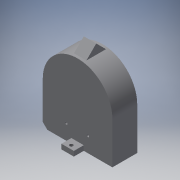
# Autodesk Inventor part: Tail2
Saved by Autodesk Inventor 2016 (Build 200138000, 138)
## iProperties
Created: 2017-03-09
Part Number: Tail2
Material: Generic
Document SubType Name: Modeling
Designer: Owner
Density: 1 g/cm^3
Appearance: Default
Author: Owner
Autodesk Inventor part; units mm, degrees
ref_plane "YZ Plane" through (0, 0, 0) normal (1, 0, 0) x (0, 1, 0)
ref_plane "XZ Plane" through (0, 0, 0) normal (0, 1, 0) x (-1, 0, 0)
sketch "Sketch1" plane through (0, 0, 0) normal (0, 0, 1) x (1, 0, 0)
  line L0 (6.35, -26.3445) -> (6.35, -31.3445) projected
  line L1 (6.35, -31.3445) -> (38.1, -31.3445) projected
  line L2 (38.1, -31.3445) -> (38.1, 11.7555) projected
  arc A0 (38.1, 11.7555) -> (-38.1, 11.7555) centre (0, 11.7555) ccw projected
  line L3 (-38.1, 11.7555) -> (-38.1, -31.3445) projected
  line L4 (-38.1, -31.3445) -> (-6.35, -31.3445) projected
  line L5 (-6.35, -31.3445) -> (-6.35, -26.3445) projected
  line L6 (-6.35, -26.3445) -> (6.35, -26.3445) projected
  circle A1 centre (0, 11.7555) radius 35.56
  line L7 (-35.56, 11.7555) -> (33.02, 11.7555)
  line L8 (33.02, -31.3445) -> (-35.56, -31.3445)
  line L9 (-35.56, -31.3445) -> (-35.56, 11.7555)
  line L10 (35.56, 11.7555) -> (-35.56, 11.7555)
  line L11 (-35.56, 11.7555) -> (-35.56, -31.3445)
  line L12 (-35.56, -31.3445) -> (35.56, -31.3445)
  line L13 (35.56, -31.3445) -> (35.56, 11.7555)
  point P0 (0, 0)
  dimension "d0" = 71.12
  constraints: 14 end point, 3 parallel, 2 horizontal, 2 point on circle, 1 centre point, 1 coincident, 1 perpendicular, 1 point on line
  measures "d0" diameter of A1
extrude "Extrusion1" add sketch "Sketch1" along normal blind 25.4 contours L6 L5 L4 L9 A1 L13 L1 L0 | L0 L8 L5 L6 | L10 L7 A1 | A1 L7 L10
sketch "Sketch2" plane through (0, 0, 0) normal (0, 0, -1) x (-1, 0, 0)
  line L0 (6.3749, -31.3445) -> (-6.9601, -31.3445) projected
  line L1 (-6.9601, -31.3445) -> (-6.9601, -26.3445) projected
  line L2 (-6.9601, -26.3445) -> (6.3749, -26.3445) projected
  line L3 (6.3749, -26.3445) -> (6.3749, -31.3445) projected
  line L4 (35.56, -31.3445) -> (-35.56, -31.3445) projected
  line L5 (0, -26.3445) -> (6.35, -26.3445)
  line L6 (6.35, -26.3445) -> (-6.35, -26.3445)
  line L7 (-6.35, -26.3445) -> (6.35, -26.3445)
  line L8 (6.35, -26.3445) -> (6.35, -21.3445)
  line L9 (6.35, -21.3445) -> (-6.35, -21.3445)
  line L10 (-6.35, -21.3445) -> (-6.35, -26.3445)
  line L11 (-6.35, -26.3445) -> (-6.35, -21.3445)
  point P0 (0, 0)
  dimension "d45" = 6.35
  dimension "d46" = 12.7
  dimension "d51" = 12.7
  constraints: 14 end point, 3 equal length, 1 horizontal, 1 perpendicular
  measures "d45" distance of L5.start L5.end
  measures "d46" distance of L5.end L6.end
  measures "d51" distance between parallel lines of L8 L10
extrude "Extrusion2" add sketch "Sketch2" along normal blind 10.16 contours L2 L10 L9 L8
sketch "Sketch4" plane through (0, 0, 25.4) normal (0, 0, 1) x (1, 0, 0)
  line L0 (-35.56, -31.3445) -> (35.56, -31.3445) projected
  line L1 (-35.56, -31.3445) -> (35.56, -31.3445)
  line L2 (0, -31.3445) -> (6.35, -31.3445)
  line L3 (6.35, -31.3445) -> (-6.35, -31.3445)
  line L4 (6.9601, -26.3445) -> (-6.35, -26.3445) projected
  line L5 (-6.35, -31.3445) -> (6.35, -31.3445)
  line L6 (6.35, -31.3445) -> (6.35, -26.3445)
  line L7 (6.35, -26.3445) -> (-6.35, -26.3445)
  line L8 (-6.35, -26.3445) -> (-6.35, -31.3445)
  point P0 (0, 0)
  dimension "d39" = 6.35
  dimension "d40" = 12.7
  dimension "d52" = 12.7
  constraints: 14 end point, 3 point on line, 2 horizontal, 2 parallel, 1 midpoint, 1 perpendicular
  measures "d39" distance of L2.start L2.end
  measures "d40" distance of L2.end L3.end
  measures "d52" distance between parallel lines of L6 L8
extrude "Extrusion4" add sketch "Sketch4" along normal blind 10.16
ref_plane "Work Plane1" through (0, -31.3445, 0) normal (-1, 0, 0) x (0, 0, 1)
sketch "Sketch7" plane through (0, -31.3445, 0) normal (-1, 0, 0) x (0, 0, 1)
  line L0 (0, 78.66) -> (0, 43.1) projected
  line L1 (0, 78.66) -> (2.7051, 78.66)
  line L2 (0, 78.66) -> (25.4, 78.66) projected
  line L3 (2.7051, 78.66) -> (22.6949, 78.66)
  line L4 (22.6949, 78.66) -> (12.6873, 78.66)
  line L5 (12.6873, 78.66) -> (12.6873, 88.6676)
  line L6 (12.6873, 88.6676) -> (22.6949, 78.66)
  line L7 (12.6873, 88.6676) -> (2.7051, 78.66)
  point P0 (0, 31.3445)
  dimension "d27" = 2.7051
  dimension "d28" = 19.9898
  dimension "d29" = 10.0076
  dimension "d30" = 10.0076
  constraints: 12 end point, 3 point on line, 1 perpendicular
  measures "d27" distance of L0.start L1.end
  measures "d28" distance of L1.end L3.end
  measures "d29" distance of L3.end L4.end
  measures "d30" distance of L4.end L5.end
extrude "Extrusion7" add sketch "Sketch7" along normal mid plane 12.7
sketch "Sketch9" plane through (-6.35, -26.3445, 25.4) normal (0, 1, 0) x (1, 0, 0)
  line L0 (12.7, -10.16) -> (0, -10.16) projected
  line L1 (6.35, -10.16) -> (6.35, -6.35)
  circle A0 centre (6.35, -6.35) radius 1.7526
  point P0 (6.35, 25.4)
  dimension "d41" = 3.81
  dimension "d42" = 3.5052
  constraints: 2 end point, 1 centre point, 1 coincident, 1 midpoint, 1 vertical
  measures "d41" distance of L1.start L1.end
  measures "d42" diameter of A0
extrude "Extrusion9" cut sketch "Sketch9" against normal blind 25.4
sketch "Sketch10" plane through (-6.35, -21.3445, 0) normal (0, 1, 0) x (1, 0, 0)
  line L0 (12.7, 10.16) -> (0, 10.16) projected
  line L1 (6.35, 10.16) -> (6.35, 6.35)
  circle A0 centre (6.35, 6.35) radius 2.2479
  point P0 (6.35, 0)
  dimension "d47" = 3.81
  dimension "d48" = 4.4958
  constraints: 2 end point, 1 centre point, 1 coincident, 1 midpoint, 1 vertical
  measures "d47" distance of L1.start L1.end
  measures "d48" diameter of A0
extrude "Extrusion10" cut sketch "Sketch10" against normal blind 25.4
sketch "Sketch11" plane through (0, 0, 0) normal (0, 0, -1) x (-1, 0, 0)
  ellipse E0 centre (-11.5997, -15.8166) end of major axis (-11.5997, -14.5666) minor radius 1.2499 projected
  ellipse E1 centre (12.5278, -15.8166) end of major axis (12.5278, -14.5666) minor radius 1.2499 projected
  line L0 (-11.5997, -15.8166) -> (-10.5997, -15.8166)
  circle A0 centre (-10.5997, -15.8166) radius 1.2446
  line L1 (12.5278, -15.8166) -> (11.5278, -15.8166)
  circle A1 centre (11.5278, -15.8166) radius 1.2446
  point P0 (0, 0)
  dimension "d53" = 1
  dimension "d54" = 2.4892
  dimension "d55" = 1
  dimension "d56" = 2.4892
  constraints: 4 end point, 2 centre point, 2 coincident, 2 horizontal, 2 other
  measures "d53" distance of L0.start L0.end
  measures "d54" diameter of A0
  measures "d55" distance of L1.start L1.end
  measures "d56" diameter of A1
extrude "Extrusion11" cut sketch "Sketch11" against normal blind 25.4 contours A0 E0 | E0 A0 | A1 E1 | E1 A1 picked at (-11.3426, -15.9919) picked at (-9.6993, -15.9182) picked at (12.2707, -15.6413) picked at (10.6274, -15.715)
body "Solid1"
